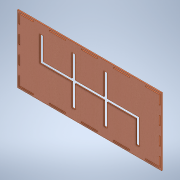
# Autodesk Inventor part: Frontal
Saved by Autodesk Inventor 2020.3 (Build 243373000, 373)
## iProperties
Created: 2020-04-04
Part Number: Frontal
Material: Madera (nogal)
Document SubType Name: Modeling
Designer: miosh
Density: 0.55 g/cm^3
Appearance: Nogal - Natural pulido
Author: miosh
Autodesk Inventor part; units mm, degrees
ref_plane "YZ Plane" through (0, 0, 0) normal (1, 0, 0) x (0, 1, 0)
ref_plane "XZ Plane" through (0, 0, 0) normal (0, 1, 0) x (-1, 0, 0)
ref_plane "XY Plane" through (0, 0, 0) normal (0, 0, 1) x (1, 0, 0)
sketch "Boceto1" plane through (0, 0, 0) normal (0, 0, 1) x (1, 0, 0)
  line L0 (0, 0) -> (0, 210)
  line L1 (0, 210) -> (450, 210)
  line L2 (450, 210) -> (450, 0)
  line L3 (450, 0) -> (0, 0)
  line L4 (0, 210) -> (5, 210)
  line L5 (5, 205) -> (50, 205)
  line L6 (50, 205) -> (50, 202)
  line L7 (5, 205) -> (5, 174.29)
  line L8 (5, 174.29) -> (8, 174.29)
  line L9 (8, 174.29) -> (8, 202)
  line L10 (8, 202) -> (50, 202)
  line L11 (0, 0) -> (5, 0)
  line L12 (0, 0) -> (5, 0)
  line L13 (5, 5) -> (50, 5)
  line L14 (5, 5) -> (5, 35.71)
  line L15 (5, 35.71) -> (8, 35.71)
  line L16 (50, 5) -> (50, 8)
  line L17 (8, 35.71) -> (8, 8)
  line L18 (8, 8) -> (50, 8)
  line L19 (450, 0) -> (445, 0)
  line L20 (445, 5) -> (445, 35.71)
  line L21 (445, 35.71) -> (442, 35.71)
  line L22 (445, 5) -> (400, 5)
  line L23 (400, 5) -> (400, 8)
  line L24 (400, 8) -> (442, 8)
  line L25 (442, 8) -> (442, 35.71)
  line L26 (450, 210) -> (445, 210)
  line L27 (445, 205) -> (400, 205)
  line L28 (445, 205) -> (445, 174.29)
  line L29 (445, 174.29) -> (442, 174.29)
  line L30 (400, 205) -> (400, 202)
  line L31 (400, 202) -> (442, 202)
  line L32 (442, 202) -> (442, 174.29)
  line L33 (5, 63.43) -> (5, 91.14)
  line L34 (5, 91.14) -> (8, 91.14)
  line L35 (8, 91.14) -> (8, 63.43)
  line L36 (8, 63.43) -> (5, 63.43)
  line L37 (5, 118.86) -> (5, 146.57)
  line L38 (5, 118.86) -> (8, 118.86)
  line L39 (8, 118.86) -> (8, 146.57)
  line L40 (8, 146.57) -> (5, 146.57)
  line L41 (445, 63.43) -> (445, 91.14)
  line L42 (445, 63.43) -> (442, 63.43)
  line L43 (442, 63.43) -> (442, 91.14)
  line L44 (442, 91.14) -> (445, 91.14)
  line L45 (445, 118.86) -> (442, 118.86)
  line L46 (442, 118.86) -> (442, 146.57)
  line L47 (442, 146.57) -> (445, 146.57)
  line L48 (445, 146.57) -> (445, 118.86)
  line L49 (350, 205) -> (300, 205)
  line L50 (300, 205) -> (300, 202)
  line L51 (300, 202) -> (350, 202)
  line L52 (350, 202) -> (350, 205)
  line L53 (250, 205) -> (200, 205)
  line L54 (200, 205) -> (200, 202)
  line L55 (200, 202) -> (250, 202)
  line L56 (250, 202) -> (250, 205)
  line L57 (150, 205) -> (100, 205)
  line L58 (100, 205) -> (100, 202)
  line L59 (100, 202) -> (150, 202)
  line L60 (150, 202) -> (150, 205)
  line L61 (350, 8) -> (300, 8)
  line L62 (300, 8) -> (300, 5)
  line L63 (300, 5) -> (350, 5)
  line L64 (350, 5) -> (350, 8)
  line L65 (250, 8) -> (200, 8)
  line L66 (200, 8) -> (200, 5)
  line L67 (200, 5) -> (250, 5)
  line L68 (250, 5) -> (250, 8)
  line L69 (150, 8) -> (100, 8)
  line L70 (100, 8) -> (100, 5)
  line L71 (100, 5) -> (150, 5)
  line L72 (150, 5) -> (150, 8)
  line L73 (450, 0) -> (450, 30)
  line L74 (380, 30) -> (380, 110)
  line L75 (380, 30) -> (370, 30)
  line L76 (370, 30) -> (370, 100)
  line L77 (380, 110) -> (280, 110)
  line L78 (370, 100) -> (280, 100)
  line L79 (280, 110) -> (280, 180)
  line L80 (280, 100) -> (280, 30)
  line L81 (280, 30) -> (270, 30)
  line L82 (270, 30) -> (270, 100)
  line L83 (280, 180) -> (270, 180)
  line L84 (270, 180) -> (270, 110)
  line L85 (270, 100) -> (180, 100)
  line L86 (270, 110) -> (180, 110)
  line L87 (180, 110) -> (180, 180)
  line L88 (180, 180) -> (170, 180)
  line L89 (170, 180) -> (170, 110)
  line L90 (180, 100) -> (180, 30)
  line L91 (180, 30) -> (170, 30)
  line L92 (170, 30) -> (170, 100)
  line L93 (170, 110) -> (80, 110)
  line L94 (80, 110) -> (80, 180)
  line L95 (80, 180) -> (70, 180)
  line L96 (70, 180) -> (70, 100)
  line L97 (70, 100) -> (170, 100)
  dimension "d93" = 450
  dimension "d94" = 210
  dimension "d95" = 210
  dimension "d96" = 450
  dimension "d97" = 5
  dimension "d98" = 30.71
  dimension "d99" = 45
  dimension "d100" = 5
  dimension "d101" = 3
  dimension "d102" = 3
  dimension "d103" = 5
  dimension "d104" = 5
  dimension "d105" = 3
  dimension "d106" = 30.71
  dimension "d107" = 45
  dimension "d108" = 3
  dimension "d109" = 5
  dimension "d110" = 30.71
  dimension "d111" = 45
  dimension "d112" = 5
  dimension "d113" = 3
  dimension "d114" = 3
  dimension "d115" = 30.71
  dimension "d116" = 5
  dimension "d117" = 45
  dimension "d118" = 5
  dimension "d119" = 3
  dimension "d120" = 3
  dimension "d121" = 3
  dimension "d122" = 3
  dimension "d123" = 3
  dimension "d124" = 5
  dimension "d125" = 5
  dimension "d126" = 5
  dimension "d127" = 5
  dimension "d128" = 5
  dimension "d129" = 5
  dimension "d130" = 27.72
  dimension "d131" = 27.71
  dimension "d132" = 27.71
  dimension "d133" = 27.72
  dimension "d134" = 27.72
  dimension "d135" = 50
  dimension "d136" = 50
  dimension "d137" = 50
  dimension "d138" = 50
  dimension "d139" = 50
  dimension "d140" = 50
  dimension "d141" = 50
  constraints: 196 end point, 43 perpendicular, 22 horizontal, 15 vertical, 6 point on line, 2 parallel, 1 collinear
  measures "d93" distance of L0.end L1.end
  measures "d94" distance of L1.end L2.end
  measures "d95" distance of L0.start L0.end
  measures "d96" distance of L2.end L0.start
  measures "d97" distance between parallel lines of L22 L3
  measures "d98" distance of L20.start L20.end
  measures "d99" distance of L20.start L22.end
  measures "d100" distance between parallel lines of L73 L20
  measures "d101" distance of L22.end L23.end
  measures "d102" distance of L20.end L21.end
  measures "d103" distance between parallel lines of L2 L28
  measures "d104" distance between parallel lines of L1 L27
  measures "d105" distance of L27.end L30.end
  measures "d106" distance of L27.start L28.end
  measures "d107" distance of L27.start L27.end
  measures "d108" distance of L28.end L29.end
  measures "d109" distance between parallel lines of L0 L7
  measures "d110" distance of L5.start L7.end
  measures "d111" distance of L5.start L5.end
  measures "d112" distance between parallel lines of L1 L5
  measures "d113" distance of L7.end L8.end
  measures "d114" distance of L5.end L6.end
  measures "d115" distance of L13.start L14.end
  measures "d116" distance between parallel lines of L0 L14
  measures "d117" distance of L13.start L13.end
  measures "d118" distance between parallel lines of L13 L3
  measures "d119" distance of L13.end L16.end
  measures "d120" distance of L14.end L15.end
  measures "d121" distance of L61.end L62.end
  measures "d122" distance of L67.end L65.start
  measures "d123" distance of L71.end L69.start
  measures "d124" distance between parallel lines of L63 L3
  measures "d125" distance between parallel lines of L3 L67
  measures "d126" distance between parallel lines of L71 L3
  measures "d127" distance between parallel lines of L1 L53
  measures "d128" distance between parallel lines of L1 L57
  measures "d129" distance between parallel lines of L1 L49
  measures "d130" distance of L14.end L33.start
  measures "d131" distance of L33.start L33.end
  measures "d132" distance of L37.start L37.end
  measures "d133" distance of L37.start L33.end
  measures "d134" distance of L37.end L7.end
  measures "d135" distance of L57.end L5.end
  measures "d136" distance of L57.start L57.end
  measures "d137" distance of L53.end L57.start
  measures "d138" distance of L53.start L53.end
  measures "d139" distance of L53.start L49.end
  measures "d140" distance of L49.start L49.end
  measures "d141" distance of L49.start L27.end
extrude "Extrusión1" add sketch "Boceto1" along normal blind 3
